Autodesk Fusion 360 part; units mm, degrees
(part 10 of 14)
  spline S90 degree 5 poles (19.8514, 6.85) (19.8445, 6.8509) (19.8307, 6.8527) (19.8101, 6.8553) (19.7826, 6.8588) (19.7482, 6.863) (19.7138, 6.867) (19.6795, 6.8709) (19.6452, 6.8747) (19.6109, 6.8783) (19.5767, 6.8818) (19.5424, 6.8852) (19.5082, 6.8884) (19.474, 6.8915) (19.4399, 6.8944) (19.4057, 6.8972) (19.3716, 6.8999) (19.3376, 6.9024) (19.3035, 6.9048) (19.2695, 6.907) (19.2355, 6.9091) (19.2015, 6.911) (19.1676, 6.9128) (19.1337, 6.9144) (19.0998, 6.9159) (19.066, 6.9173) (19.0322, 6.9185) (18.9984, 6.9195) (18.9647, 6.9204) (18.931, 6.9211) (18.8973, 6.9217) (18.8637, 6.9221) (18.8301, 6.9224) (18.7966, 6.9224) (18.7631, 6.9224) (18.7296, 6.9221) (18.6962, 6.9218) (18.6628, 6.9212) (18.6294, 6.9205) (18.5961, 6.9195) (18.5629, 6.9185) (18.5296, 6.9172) (18.4965, 6.9158) (18.4634, 6.9142) (18.4303, 6.9124) (18.3973, 6.9104) (18.3643, 6.9083) (18.3314, 6.9059) (18.2985, 6.9033) (18.2657, 6.9006) (18.233, 6.8977) (18.2003, 6.8945) (18.1676, 6.8912) (18.1351, 6.8876) (18.1026, 6.8838) (18.0701, 6.8798) (18.0378, 6.8756) (18.0101, 6.8717) (17.9889, 6.8687) (17.9742, 6.8665) (17.9659, 6.8652) (17.9641, 6.8649) knots -1 -1 -1 -1 -1 -1 -0.985714 -0.971429 -0.957143 -0.942857 -0.928571 -0.914286 -0.9 -0.885714 -0.871429 -0.857143 -0.842857 -0.828571 -0.814286 -0.8 -0.785714 -0.771429 -0.757143 -0.742857 -0.728571 -0.714286 -0.7 -0.685714 -0.671429 -0.657143 -0.642857 -0.628571 -0.614286 -0.6 -0.585714 -0.571429 -0.557143 -0.542857 -0.528571 -0.514286 -0.5 -0.485714 -0.471429 -0.457143 -0.442857 -0.428571 -0.414286 -0.4 -0.385714 -0.371429 -0.357143 -0.342857 -0.328571 -0.314286 -0.3 -0.285714 -0.271429 -0.257143 -0.242857 -0.228571 -0.214286 -0.2 -0.195913 -0.195913 -0.195913 -0.195913 -0.195913 -0.195913
  spline S91 degree 3 poles (17.426, 7.1689) (17.4508, 7.1087) (17.4871, 7.0539) (17.5786, 6.9613) (17.633, 6.9244) (17.7354, 6.8809) (17.7803, 6.8688) (17.872, 6.8573) (17.9184, 6.8579) (17.9641, 6.8649) knots 0 0 0 0 0.019532 0.019532 0.039064 0.039064 0.052927 0.052927 0.06679 0.06679 0.06679 0.06679
  arc A46 (17.426, 7.1689) -> (17.3912, 7.2528) centre (0, 0) ccw
  spline S92 degree 3 poles (17.5567, 7.8483) (17.5043, 7.8098) (17.4598, 7.7613) (17.392, 7.6502) (17.3693, 7.5885) (17.3517, 7.4786) (17.3507, 7.4322) (17.3617, 7.3404) (17.3734, 7.2955) (17.3912, 7.2528) knots 0 0 0 0 0.019532 0.019532 0.039064 0.039064 0.052927 0.052927 0.06679 0.06679 0.06679 0.06679
  spline S93 degree 5 poles (17.5567, 7.8483) (17.5582, 7.8494) (17.565, 7.8544) (17.577, 7.8632) (17.5941, 7.876) (17.6164, 7.8929) (17.6423, 7.9127) (17.668, 7.9329) (17.6937, 7.9532) (17.7192, 7.9737) (17.7447, 7.9944) (17.77, 8.0153) (17.7953, 8.0364) (17.8204, 8.0576) (17.8455, 8.079) (17.8704, 8.1006) (17.8952, 8.1224) (17.92, 8.1444) (17.9446, 8.1665) (17.9692, 8.1888) (17.9936, 8.2112) (18.018, 8.2338) (18.0423, 8.2566) (18.0665, 8.2795) (18.0906, 8.3026) (18.1146, 8.3258) (18.1385, 8.3491) (18.1623, 8.3726) (18.1861, 8.3963) (18.2098, 8.4201) (18.2333, 8.444) (18.2568, 8.4681) (18.2802, 8.4923) (18.3035, 8.5166) (18.3267, 8.5411) (18.3499, 8.5657) (18.3729, 8.5905) (18.3959, 8.6153) (18.4188, 8.6403) (18.4416, 8.6655) (18.4644, 8.6907) (18.487, 8.7161) (18.5096, 8.7416) (18.532, 8.7672) (18.5544, 8.793) (18.5768, 8.8189) (18.599, 8.8449) (18.6211, 8.871) (18.6432, 8.8972) (18.6652, 8.9236) (18.6871, 8.95) (18.709, 8.9766) (18.7307, 9.0033) (18.7524, 9.0301) (18.774, 9.0571) (18.7955, 9.0841) (18.8169, 9.1112) (18.8383, 9.1385) (18.8553, 9.1604) (18.868, 9.1769) (18.8765, 9.1879) (18.8807, 9.1934) knots 0.195913 0.195913 0.195913 0.195913 0.195913 0.195913 0.2 0.214286 0.228571 0.242857 0.257143 0.271429 0.285714 0.3 0.314286 0.328571 0.342857 0.357143 0.371429 0.385714 0.4 0.414286 0.428571 0.442857 0.457143 0.471429 0.485714 0.5 0.514286 0.528571 0.542857 0.557143 0.571429 0.585714 0.6 0.614286 0.628571 0.642857 0.657143 0.671429 0.685714 0.7 0.714286 0.728571 0.742857 0.757143 0.771429 0.785714 0.8 0.814286 0.828571 0.842857 0.857143 0.871429 0.885714 0.9 0.914286 0.928571 0.942857 0.957143 0.971429 0.985714 1 1 1 1 1 1
  arc A47 (18.8807, 9.1934) -> (18.5354, 9.8711) centre (0, 0) ccw
  spline S94 degree 5 poles (18.5354, 9.8711) (18.5285, 9.8709) (18.5146, 9.8705) (18.4938, 9.8699) (18.4661, 9.869) (18.4315, 9.8678) (18.3969, 9.8664) (18.3624, 9.8649) (18.3279, 9.8632) (18.2935, 9.8614) (18.2591, 9.8595) (18.2247, 9.8575) (18.1905, 9.8553) (18.1562, 9.853) (18.122, 9.8506) (18.0879, 9.848) (18.0538, 9.8453) (18.0197, 9.8425) (17.9857, 9.8395) (17.9518, 9.8364) (17.9179, 9.8331) (17.884, 9.8297) (17.8502, 9.8262) (17.8165, 9.8225) (17.7828, 9.8187) (17.7492, 9.8147) (17.7156, 9.8106) (17.6821, 9.8063) (17.6486, 9.8019) (17.6152, 9.7974) (17.5819, 9.7927) (17.5486, 9.7878) (17.5154, 9.7828) (17.4822, 9.7777) (17.4492, 9.7723) (17.4161, 9.7669) (17.3832, 9.7613) (17.3503, 9.7555) (17.3175, 9.7495) (17.2847, 9.7434) (17.252, 9.7372) (17.2194, 9.7307) (17.1869, 9.7241) (17.1544, 9.7174) (17.122, 9.7104) (17.0897, 9.7033) (17.0575, 9.696) (17.0254, 9.6885) (16.9933, 9.6809) (16.9613, 9.673) (16.9295, 9.665) (16.8977, 9.6568) (16.866, 9.6484) (16.8343, 9.6397) (16.8028, 9.6309) (16.7714, 9.6219) (16.7401, 9.6127) (16.7134, 9.6045) (16.6929, 9.5982) (16.6788, 9.5937) (16.6708, 9.5912) (16.669, 9.5906) knots -1 -1 -1 -1 -1 -1 -0.985714 -0.971429 -0.957143 -0.942857 -0.928571 -0.914286 -0.9 -0.885714 -0.871429 -0.857143 -0.842857 -0.828571 -0.814286 -0.8 -0.785714 -0.771429 -0.757143 -0.742857 -0.728571 -0.714286 -0.7 -0.685714 -0.671429 -0.657143 -0.642857 -0.628571 -0.614286 -0.6 -0.585714 -0.571429 -0.557143 -0.542857 -0.528571 -0.514286 -0.5 -0.485714 -0.471429 -0.457143 -0.442857 -0.428571 -0.414286 -0.4 -0.385714 -0.371429 -0.357143 -0.342857 -0.328571 -0.314286 -0.3 -0.285714 -0.271429 -0.257143 -0.242857 -0.228571 -0.214286 -0.2 -0.195913 -0.195913 -0.195913 -0.195913 -0.195913 -0.195913
  spline S95 degree 3 poles (16.09, 9.8067) (16.1239, 9.7511) (16.1683, 9.7026) (16.2732, 9.6255) (16.3327, 9.5976) (16.4407, 9.5706) (16.4869, 9.5657) (16.5792, 9.5687) (16.625, 9.5765) (16.669, 9.5906) knots 0 0 0 0 0.019532 0.019532 0.039064 0.039064 0.052927 0.052927 0.06679 0.06679 0.06679 0.06679
  arc A48 (16.09, 9.8067) -> (16.0425, 9.8841) centre (0, 0) ccw
  spline S96 degree 3 poles (16.1129, 10.4982) (16.067, 10.4519) (16.0307, 10.3971) (15.9811, 10.2767) (15.9683, 10.2122) (15.9681, 10.1009) (15.9745, 10.0549) (15.9996, 9.966) (16.0183, 9.9235) (16.0425, 9.8841) knots 0 0 0 0 0.019532 0.019532 0.039064 0.039064 0.052927 0.052927 0.06679 0.06679 0.06679 0.06679
  spline S97 degree 5 poles (16.1129, 10.4982) (16.1142, 10.4995) (16.12, 10.5054) (16.1305, 10.516) (16.1454, 10.5314) (16.1648, 10.5515) (16.1872, 10.5752) (16.2096, 10.5991) (16.2317, 10.6232) (16.2537, 10.6474) (16.2756, 10.6718) (16.2974, 10.6964) (16.319, 10.7212) (16.3405, 10.7461) (16.3619, 10.7712) (16.3832, 10.7965) (16.4043, 10.8219) (16.4253, 10.8474) (16.4462, 10.8731) (16.4669, 10.899) (16.4876, 10.925) (16.5081, 10.9511) (16.5286, 10.9774) (16.5489, 11.0038) (16.5691, 11.0303) (16.5891, 11.057) (16.6091, 11.0838) (16.629, 11.1108) (16.6487, 11.1378) (16.6684, 11.165) (16.6879, 11.1924) (16.7073, 11.2198) (16.7267, 11.2474) (16.7459, 11.2751) (16.765, 11.3029) (16.784, 11.3308) (16.8029, 11.3589) (16.8217, 11.387) (16.8404, 11.4153) (16.859, 11.4437) (16.8775, 11.4722) (16.8959, 11.5008) (16.9142, 11.5295) (16.9324, 11.5584) (16.9505, 11.5873) (16.9685, 11.6163) (16.9864, 11.6455) (17.0042, 11.6748) (17.0219, 11.7041) (17.0395, 11.7336) (17.057, 11.7632) (17.0744, 11.7928) (17.0917, 11.8226) (17.1089, 11.8525) (17.126, 11.8824) (17.143, 11.9125) (17.1599, 11.9427) (17.1768, 11.9729) (17.1902, 11.9972) (17.2001, 12.0155) (17.2068, 12.0277) (17.2101, 12.0338) knots 0.195913 0.195913 0.195913 0.195913 0.195913 0.195913 0.2 0.214286 0.228571 0.242857 0.257143 0.271429 0.285714 0.3 0.314286 0.328571 0.342857 0.357143 0.371429 0.385714 0.4 0.414286 0.428571 0.442857 0.457143 0.471429 0.485714 0.5 0.514286 0.528571 0.542857 0.557143 0.571429 0.585714 0.6 0.614286 0.628571 0.642857 0.657143 0.671429 0.685714 0.7 0.714286 0.728571 0.742857 0.757143 0.771429 0.785714 0.8 0.814286 0.828571 0.842857 0.857143 0.871429 0.885714 0.9 0.914286 0.928571 0.942857 0.957143 0.971429 0.985714 1 1 1 1 1 1
  arc A49 (17.2101, 12.0338) -> (16.763, 12.6491) centre (0, 0) ccw
  spline S98 degree 5 poles (16.763, 12.6491) (16.7562, 12.6479) (16.7426, 12.6453) (16.7221, 12.6415) (16.6949, 12.6362) (16.6609, 12.6296) (16.627, 12.6228) (16.5931, 12.6159) (16.5593, 12.6089) (16.5256, 12.6018) (16.4919, 12.5945) (16.4583, 12.5871) (16.4248, 12.5796) (16.3913, 12.572) (16.3579, 12.5642) (16.3246, 12.5563) (16.2913, 12.5483) (16.2582, 12.5402) (16.225, 12.5319) (16.192, 12.5235) (16.159, 12.515) (16.1261, 12.5064) (16.0933, 12.4976) (16.0606, 12.4887) (16.0279, 12.4796) (15.9953, 12.4704) (15.9628, 12.4611) (15.9303, 12.4517) (15.898, 12.4421) (15.8657, 12.4324) (15.8335, 12.4225) (15.8014, 12.4125) (15.7694, 12.4024) (15.7374, 12.3921) (15.7056, 12.3817) (15.6738, 12.3711) (15.6422, 12.3604) (15.6106, 12.3496) (15.5791, 12.3385) (15.5477, 12.3274) (15.5164, 12.3161) (15.4852, 12.3046) (15.4541, 12.293) (15.4231, 12.2813) (15.3922, 12.2693) (15.3614, 12.2573) (15.3307, 12.245) (15.3001, 12.2326) (15.2697, 12.22) (15.2393, 12.2073) (15.2091, 12.1944) (15.179, 12.1813) (15.149, 12.168) (15.1191, 12.1545) (15.0894, 12.1409) (15.0597, 12.1271) (15.0303, 12.113) (15.0051, 12.1008) (14.9859, 12.0914) (14.9726, 12.0847) (14.9651, 12.081) (14.9635, 12.0801) knots -1 -1 -1 -1 -1 -1 -0.985714 -0.971429 -0.957143 -0.942857 -0.928571 -0.914286 -0.9 -0.885714 -0.871429 -0.857143 -0.842857 -0.828571 -0.814286 -0.8 -0.785714 -0.771429 -0.757143 -0.742857 -0.728571 -0.714286 -0.7 -0.685714 -0.671429 -0.657143 -0.642857 -0.628571 -0.614286 -0.6 -0.585714 -0.571429 -0.557143 -0.542857 -0.528571 -0.514286 -0.5 -0.485714 -0.471429 -0.457143 -0.442857 -0.428571 -0.414286 -0.4 -0.385714 -0.371429 -0.357143 -0.342857 -0.328571 -0.314286 -0.3 -0.285714 -0.271429 -0.257143 -0.242857 -0.228571 -0.214286 -0.2 -0.195913 -0.195913 -0.195913 -0.195913 -0.195913 -0.195913
  spline S99 degree 3 poles (14.3578, 12.203) (14.4, 12.1534) (14.4514, 12.1125) (14.5671, 12.0527) (14.6302, 12.0344) (14.7411, 12.0247) (14.7875, 12.027) (14.8782, 12.0444) (14.9222, 12.0594) (14.9635, 12.0801) knots 0 0 0 0 0.019532 0.019532 0.039064 0.039064 0.052927 0.052927 0.06679 0.06679 0.06679 0.06679
  arc A50 (14.3578, 12.203) -> (14.2988, 12.2721) centre (0, 0) ccw
  spline S100 degree 3 poles (14.2722, 12.8895) (14.2342, 12.8366) (14.2069, 12.7769) (14.1767, 12.6502) (14.1742, 12.5845) (14.1914, 12.4745) (14.2049, 12.4301) (14.2436, 12.3462) (14.2687, 12.3071) (14.2988, 12.2721) knots 0 0 0 0 0.019532 0.019532 0.039064 0.039064 0.052927 0.052927 0.06679 0.06679 0.06679 0.06679
  spline S101 degree 5 poles (14.2722, 12.8895) (14.2733, 12.891) (14.2782, 12.8978) (14.2868, 12.9099) (14.2992, 12.9274) (14.3152, 12.9503) (14.3336, 12.9772) (14.3519, 13.0043) (14.37, 13.0316) (14.388, 13.059) (14.4058, 13.0865) (14.4234, 13.1142) (14.4409, 13.1421) (14.4583, 13.17) (14.4755, 13.1982) (14.4925, 13.2264) (14.5094, 13.2548) (14.5262, 13.2833) (14.5428, 13.312) (14.5592, 13.3408) (14.5756, 13.3697) (14.5918, 13.3987) (14.6078, 13.4279) (14.6237, 13.4571) (14.6395, 13.4865) (14.6552, 13.516) (14.6707, 13.5456) (14.6861, 13.5753) (14.7014, 13.6051) (14.7166, 13.6351) (14.7316, 13.6651) (14.7465, 13.6953) (14.7612, 13.7255) (14.7759, 13.7559) (14.7904, 13.7863) (14.8048, 13.8169) (14.8191, 13.8476) (14.8333, 13.8783) (14.8473, 13.9092) (14.8613, 13.9401) (14.8751, 13.9712) (14.8888, 14.0023) (14.9023, 14.0335) (14.9158, 14.0649) (14.9291, 14.0963) (14.9424, 14.1278) (14.9555, 14.1594) (14.9685, 14.1911) (14.9814, 14.2228) (14.9941, 14.2547) (15.0068, 14.2866) (15.0193, 14.3187) (15.0318, 14.3508) (15.0441, 14.383) (15.0563, 14.4152) (15.0684, 14.4476) (15.0804, 14.4801) (15.0923, 14.5126) (15.1017, 14.5387) (15.1087, 14.5583) (15.1134, 14.5713) (15.1157, 14.5779) knots 0.195913 0.195913 0.195913 0.195913 0.195913 0.195913 0.2 0.214286 0.228571 0.242857 0.257143 0.271429 0.285714 0.3 0.314286 0.328571 0.342857 0.357143 0.371429 0.385714 0.4 0.414286 0.428571 0.442857 0.457143 0.471429 0.485714 0.5 0.514286 0.528571 0.542857 0.557143 0.571429 0.585714 0.6 0.614286 0.628571 0.642857 0.657143 0.671429 0.685714 0.7 0.714286 0.728571 0.742857 0.757143 0.771429 0.785714 0.8 0.814286 0.828571 0.842857 0.857143 0.871429 0.885714 0.9 0.914286 0.928571 0.942857 0.957143 0.971429 0.985714 1 1 1 1 1 1
  arc A51 (15.1157, 14.5779) -> (14.5779, 15.1157) centre (0, 0) ccw
  spline S102 degree 5 poles (14.5779, 15.1157) (14.5713, 15.1134) (14.5583, 15.1087) (14.5387, 15.1017) (14.5126, 15.0923) (14.4801, 15.0804) (14.4476, 15.0684) (14.4152, 15.0563) (14.383, 15.0441) (14.3508, 15.0318) (14.3187, 15.0193) (14.2866, 15.0068) (14.2547, 14.9941) (14.2228, 14.9814) (14.1911, 14.9685) (14.1594, 14.9555) (14.1278, 14.9424) (14.0963, 14.9291) (14.0649, 14.9158) (14.0335, 14.9023) (14.0023, 14.8888) (13.9712, 14.8751) (13.9401, 14.8613) (13.9092, 14.8473) (13.8783, 14.8333) (13.8476, 14.8191) (13.8169, 14.8048) (13.7863, 14.7904) (13.7559, 14.7759) (13.7255, 14.7612) (13.6953, 14.7465) (13.6651, 14.7316) (13.6351, 14.7166) (13.6051, 14.7014) (13.5753, 14.6861) (13.5456, 14.6707) (13.516, 14.6552) (13.4865, 14.6395) (13.4571, 14.6237) (13.4279, 14.6078) (13.3987, 14.5918) (13.3697, 14.5756) (13.3408, 14.5592) (13.312, 14.5428) (13.2833, 14.5262) (13.2548, 14.5094) (13.2264, 14.4925) (13.1982, 14.4755) (13.17, 14.4583) (13.1421, 14.4409) (13.1142, 14.4234) (13.0865, 14.4058) (13.059, 14.388) (13.0316, 14.37) (13.0043, 14.3519) (12.9772, 14.3336) (12.9503, 14.3152) (12.9274, 14.2992) (12.9099, 14.2868) (12.8978, 14.2782) (12.891, 14.2733) (12.8895, 14.2722) knots -1 -1 -1 -1 -1 -1 -0.985714 -0.971429 -0.957143 -0.942857 -0.928571 -0.914286 -0.9 -0.885714 -0.871429 -0.857143 -0.842857 -0.828571 -0.814286 -0.8 -0.785714 -0.771429 -0.757143 -0.742857 -0.728571 -0.714286 -0.7 -0.685714 -0.671429 -0.657143 -0.642857 -0.628571 -0.614286 -0.6 -0.585714 -0.571429 -0.557143 -0.542857 -0.528571 -0.514286 -0.5 -0.485714 -0.471429 -0.457143 -0.442857 -0.428571 -0.414286 -0.4 -0.385714 -0.371429 -0.357143 -0.342857 -0.328571 -0.314286 -0.3 -0.285714 -0.271429 -0.257143 -0.242857 -0.228571 -0.214286 -0.2 -0.195913 -0.195913 -0.195913 -0.195913 -0.195913 -0.195913
  spline S103 degree 3 poles (12.2721, 14.2988) (12.3215, 14.2564) (12.3787, 14.224) (12.5023, 14.1831) (12.5675, 14.1749) (12.6785, 14.1826) (12.724, 14.1922) (12.8109, 14.2236) (12.852, 14.2452) (12.8895, 14.2722) knots 0 0 0 0 0.019532 0.019532 0.039064 0.039064 0.052927 0.052927 0.06679 0.06679 0.06679 0.06679
  arc A52 (12.2721, 14.2988) -> (12.203, 14.3578) centre (0, 0) ccw
  spline S104 degree 3 poles (12.0801, 14.9635) (12.0509, 14.9053) (12.0332, 14.842) (12.0233, 14.7122) (12.031, 14.6469) (12.0652, 14.541) (12.0855, 14.4992) (12.1369, 14.4224) (12.1678, 14.3877) (12.203, 14.3578) knots 0 0 0 0 0.019532 0.019532 0.039064 0.039064 0.052927 0.052927 0.06679 0.06679 0.06679 0.06679
  spline S105 degree 5 poles (12.0801, 14.9635) (12.081, 14.9651) (12.0847, 14.9726) (12.0914, 14.9859) (12.1008, 15.0051) (12.113, 15.0303) (12.1271, 15.0597) (12.1409, 15.0894) (12.1545, 15.1191) (12.168, 15.149) (12.1813, 15.179) (12.1944, 15.2091) (12.2073, 15.2393) (12.22, 15.2697) (12.2326, 15.3001) (12.245, 15.3307) (12.2573, 15.3614) (12.2693, 15.3922) (12.2813, 15.4231) (12.293, 15.4541) (12.3046, 15.4852) (12.3161, 15.5164) (12.3274, 15.5477) (12.3385, 15.5791) (12.3496, 15.6106) (12.3604, 15.6422) (12.3711, 15.6738) (12.3817, 15.7056) (12.3921, 15.7374) (12.4024, 15.7694) (12.4125, 15.8014) (12.4225, 15.8335) (12.4324, 15.8657) (12.4421, 15.898) (12.4517, 15.9303) (12.4611, 15.9628) (12.4704, 15.9953) (12.4796, 16.0279) (12.4887, 16.0606) (12.4976, 16.0933) (12.5064, 16.1261) (12.515, 16.159) (12.5235, 16.192) (12.5319, 16.225) (12.5402, 16.2582) (12.5483, 16.2913) (12.5563, 16.3246) (12.5642, 16.3579) (12.572, 16.3913) (12.5796, 16.4248) (12.5871, 16.4583) (12.5945, 16.4919) (12.6018, 16.5256) (12.6089, 16.5593) (12.6159, 16.5931) (12.6228, 16.627) (12.6296, 16.6609) (12.6362, 16.6949) (12.6415, 16.7221) (12.6453, 16.7426) (12.6479, 16.7562) (12.6491, 16.763) knots 0.195913 0.195913 0.195913 0.195913 0.195913 0.195913 0.2 0.214286 0.228571 0.242857 0.257143 0.271429 0.285714 0.3 0.314286 0.328571 0.342857 0.357143 0.371429 0.385714 0.4 0.414286 0.428571 0.442857 0.457143 0.471429 0.485714 0.5 0.514286 0.528571 0.542857 0.557143 0.571429 0.585714 0.6 0.614286 0.628571 0.642857 0.657143 0.671429 0.685714 0.7 0.714286 0.728571 0.742857 0.757143 0.771429 0.785714 0.8 0.814286 0.828571 0.842857 0.857143 0.871429 0.885714 0.9 0.914286 0.928571 0.942857 0.957143 0.971429 0.985714 1 1 1 1 1 1
  arc A53 (12.6491, 16.763) -> (12.0338, 17.2101) centre (0, 0) ccw
  spline S106 degree 5 poles (12.0338, 17.2101) (12.0277, 17.2068) (12.0155, 17.2001) (11.9972, 17.1902) (11.9729, 17.1768) (11.9427, 17.1599) (11.9125, 17.143) (11.8824, 17.126) (11.8525, 17.1089) (11.8226, 17.0917) (11.7928, 17.0744) (11.7632, 17.057) (11.7336, 17.0395) (11.7041, 17.0219) (11.6748, 17.0042) (11.6455, 16.9864) (11.6163, 16.9685) (11.5873, 16.9505) (11.5584, 16.9324) (11.5295, 16.9142) (11.5008, 16.8959) (11.4722, 16.8775) (11.4437, 16.859) (11.4153, 16.8404) (11.387, 16.8217) (11.3589, 16.8029) (11.3308, 16.784) (11.3029, 16.765) (11.2751, 16.7459) (11.2474, 16.7267) (11.2198, 16.7073) (11.1924, 16.6879) (11.165, 16.6684) (11.1378, 16.6487) (11.1108, 16.629) (11.0838, 16.6091) (11.057, 16.5891) (11.0303, 16.5691) (11.0038, 16.5489) (10.9774, 16.5286) (10.9511, 16.5081) (10.925, 16.4876) (10.899, 16.4669) (10.8731, 16.4462) (10.8474, 16.4253) (10.8219, 16.4043) (10.7965, 16.3832) (10.7712, 16.3619) (10.7461, 16.3405) (10.7212, 16.319) (10.6964, 16.2974) (10.6718, 16.2756) (10.6474, 16.2537) (10.6232, 16.2317) (10.5991, 16.2096) (10.5752, 16.1872) (10.5515, 16.1648) (10.5314, 16.1454) (10.516, 16.1305) (10.5054, 16.12) (10.4995, 16.1142) (10.4982, 16.1129) knots -1 -1 -1 -1 -1 -1 -0.985714 -0.971429 -0.957143 -0.942857 -0.928571 -0.914286 -0.9 -0.885714 -0.871429 -0.857143 -0.842857 -0.828571 -0.814286 -0.8 -0.785714 -0.771429 -0.757143 -0.742857 -0.728571 -0.714286 -0.7 -0.685714 -0.671429 -0.657143 -0.642857 -0.628571 -0.614286 -0.6 -0.585714 -0.571429 -0.557143 -0.542857 -0.528571 -0.514286 -0.5 -0.485714 -0.471429 -0.457143 -0.442857 -0.428571 -0.414286 -0.4 -0.385714 -0.371429 -0.357143 -0.342857 -0.328571 -0.314286 -0.3 -0.285714 -0.271429 -0.257143 -0.242857 -0.228571 -0.214286 -0.2 -0.195913 -0.195913 -0.195913 -0.195913 -0.195913 -0.195913
  spline S107 degree 3 poles (9.8841, 16.0425) (9.9396, 16.0084) (10.0011, 15.9854) (10.1296, 15.9643) (10.1953, 15.9664) (10.3038, 15.9914) (10.3472, 16.008) (10.4281, 16.0525) (10.4653, 16.0803) (10.4982, 16.1129) knots 0 0 0 0 0.019532 0.019532 0.039064 0.039064 0.052927 0.052927 0.06679 0.06679 0.06679 0.06679
  arc A54 (9.8841, 16.0425) -> (9.8067, 16.09) centre (0, 0) ccw
  spline S108 degree 3 poles (9.5906, 16.669) (9.5708, 16.607) (9.5633, 16.5417) (9.5737, 16.4119) (9.5916, 16.3486) (9.642, 16.2494) (9.6685, 16.2113) (9.7313, 16.1434) (9.7672, 16.114) (9.8067, 16.09) knots 0 0 0 0 0.019532 0.019532 0.039064 0.039064 0.052927 0.052927 0.06679 0.06679 0.06679 0.06679
  spline S109 degree 5 poles (9.5906, 16.669) (9.5912, 16.6708) (9.5937, 16.6788) (9.5982, 16.6929) (9.6045, 16.7134) (9.6127, 16.7401) (9.6219, 16.7714) (9.6309, 16.8028) (9.6397, 16.8343) (9.6484, 16.866) (9.6568, 16.8977) (9.665, 16.9295) (9.673, 16.9613) (9.6809, 16.9933) (9.6885, 17.0254) (9.696, 17.0575) (9.7033, 17.0897) (9.7104, 17.122) (9.7174, 17.1544) (9.7241, 17.1869) (9.7307, 17.2194) (9.7372, 17.252) (9.7434, 17.2847) (9.7495, 17.3175) (9.7555, 17.3503) (9.7613, 17.3832) (9.7669, 17.4161) (9.7723, 17.4492) (9.7777, 17.4822) (9.7828, 17.5154) (9.7878, 17.5486) (9.7927, 17.5819) (9.7974, 17.6152) (9.8019, 17.6486) (9.8063, 17.6821) (9.8106, 17.7156) (9.8147, 17.7492) (9.8187, 17.7828) (9.8225, 17.8165) (9.8262, 17.8502) (9.8297, 17.884) (9.8331, 17.9179) (9.8364, 17.9518) (9.8395, 17.9857) (9.8425, 18.0197) (9.8453, 18.0538) (9.848, 18.0879) (9.8506, 18.122) (9.853, 18.1562) (9.8553, 18.1905) (9.8575, 18.2247) (9.8595, 18.2591) (9.8614, 18.2935) (9.8632, 18.3279) (9.8649, 18.3624) (9.8664, 18.3969) (9.8678, 18.4315) (9.869, 18.4661) (9.8699, 18.4938) (9.8705, 18.5146) (9.8709, 18.5285) (9.8711, 18.5354) knots 0.195913 0.195913 0.195913 0.195913 0.195913 0.195913 0.2 0.214286 0.228571 0.242857 0.257143 0.271429 0.285714 0.3 0.314286 0.328571 0.342857 0.357143 0.371429 0.385714 0.4 0.414286 0.428571 0.442857 0.457143 0.471429 0.485714 0.5 0.514286 0.528571 0.542857 0.557143 0.571429 0.585714 0.6 0.614286 0.628571 0.642857 0.657143 0.671429 0.685714 0.7 0.714286 0.728571 0.742857 0.757143 0.771429 0.785714 0.8 0.814286 0.828571 0.842857 0.857143 0.871429 0.885714 0.9 0.914286 0.928571 0.942857 0.957143 0.971429 0.985714 1 1 1 1 1 1
  arc A55 (9.8711, 18.5354) -> (9.1934, 18.8807) centre (0, 0) ccw
  spline S110 degree 5 poles (9.1934, 18.8807) (9.1879, 18.8765) (9.1769, 18.868) (9.1604, 18.8553) (9.1385, 18.8383) (9.1112, 18.8169) (9.0841, 18.7955) (9.0571, 18.774) (9.0301, 18.7524) (9.0033, 18.7307) (8.9766, 18.709) (8.95, 18.6871) (8.9236, 18.6652) (8.8972, 18.6432) (8.871, 18.6211) (8.8449, 18.599) (8.8189, 18.5768) (8.793, 18.5544) (8.7672, 18.532) (8.7416, 18.5096) (8.7161, 18.487) (8.6907, 18.4644) (8.6655, 18.4416) (8.6403, 18.4188) (8.6153, 18.3959) (8.5905, 18.3729) (8.5657, 18.3499) (8.5411, 18.3267) (8.5166, 18.3035) (8.4923, 18.2802) (8.4681, 18.2568) (8.444, 18.2333) (8.4201, 18.2098) (8.3963, 18.1861) (8.3726, 18.1623) (8.3491, 18.1385) (8.3258, 18.1146) (8.3026, 18.0906) (8.2795, 18.0665) (8.2566, 18.0423) (8.2338, 18.018) (8.2112, 17.9936) (8.1888, 17.9692) (8.1665, 17.9446) (8.1444, 17.92) (8.1224, 17.8952) (8.1006, 17.8704) (8.079, 17.8455) (8.0576, 17.8204) (8.0364, 17.7953) (8.0153, 17.77) (7.9944, 17.7447) (7.9737, 17.7192) (7.9532, 17.6937) (7.9329, 17.668) (7.9127, 17.6423) (7.8929, 17.6164) (7.876, 17.5941) (7.8632, 17.577) (7.8544, 17.565) (7.8494, 17.5582) (7.8483, 17.5567) knots -1 -1 -1 -1 -1 -1 -0.985714 -0.971429 -0.957143 -0.942857 -0.928571 -0.914286 -0.9 -0.885714 -0.871429 -0.857143 -0.842857 -0.828571 -0.814286 -0.8 -0.785714 -0.771429 -0.757143 -0.742857 -0.728571 -0.714286 -0.7 -0.685714 -0.671429 -0.657143 -0.642857 -0.628571 -0.614286 -0.6 -0.585714 -0.571429 -0.557143 -0.542857 -0.528571 -0.514286 -0.5 -0.485714 -0.471429 -0.457143 -0.442857 -0.428571 -0.414286 -0.4 -0.385714 -0.371429 -0.357143 -0.342857 -0.328571 -0.314286 -0.3 -0.285714 -0.271429 -0.257143 -0.242857 -0.228571 -0.214286 -0.2 -0.195913 -0.195913 -0.195913 -0.195913 -0.195913 -0.195913
  spline S111 degree 3 poles (7.2528, 17.3912) (7.3129, 17.3662) (7.3774, 17.3531) (7.5076, 17.3523) (7.5721, 17.3647) (7.6753, 17.4064) (7.7156, 17.4295) (7.7886, 17.4862) (7.821, 17.5195) (7.8483, 17.5567) knots 0 0 0 0 0.019532 0.019532 0.039064 0.039064 0.052927 0.052927 0.06679 0.06679 0.06679 0.06679
  arc A56 (7.2528, 17.3912) -> (7.1689, 17.426) centre (0, 0) ccw
  spline S112 degree 3 poles (6.8649, 17.9641) (6.8551, 17.8997) (6.8579, 17.8341) (6.8885, 17.7075) (6.916, 17.6478) (6.9813, 17.5577) (7.0135, 17.5242) (7.0861, 17.467) (7.1262, 17.4436) (7.1689, 17.426) knots 0 0 0 0 0.019532 0.019532 0.039064 0.039064 0.052927 0.052927 0.06679 0.06679 0.06679 0.06679
  spline S113 degree 5 poles (6.8649, 17.9641) (6.8652, 17.9659) (6.8665, 17.9742) (6.8687, 17.9889) (6.8717, 18.0101) (6.8756, 18.0378) (6.8798, 18.0701) (6.8838, 18.1026) (6.8876, 18.1351) (6.8912, 18.1676) (6.8945, 18.2003) (6.8977, 18.233) (6.9006, 18.2657) (6.9033, 18.2985) (6.9059, 18.3314) (6.9083, 18.3643) (6.9104, 18.3973) (6.9124, 18.4303) (6.9142, 18.4634) (6.9158, 18.4965) (6.9172, 18.5296) (6.9185, 18.5629) (6.9195, 18.5961) (6.9205, 18.6294) (6.9212, 18.6628) (6.9218, 18.6962) (6.9221, 18.7296) (6.9224, 18.7631) (6.9224, 18.7966) (6.9224, 18.8301) (6.9221, 18.8637) (6.9217, 18.8973) (6.9211, 18.931) (6.9204, 18.9647) (6.9195, 18.9984) (6.9185, 19.0322) (6.9173, 19.066) (6.9159, 19.0998) (6.9144, 19.1337) (6.9128, 19.1676) (6.911, 19.2015) (6.9091, 19.2355) (6.907, 19.2695) (6.9048, 19.3035) (6.9024, 19.3376) (6.8999, 19.3716) (6.8972, 19.4057) (6.8944, 19.4399) (6.8915, 19.474) (6.8884, 19.5082) (6.8852, 19.5424) (6.8818, 19.5767) (6.8783, 19.6109) (6.8747, 19.6452) (6.8709, 19.6795) (6.867, 19.7138) (6.863, 19.7482) (6.8588, 19.7826) (6.8553, 19.8101) (6.8527, 19.8307) (6.8509, 19.8445) (6.85, 19.8514) knots 0.195913 0.195913 0.195913 0.195913 0.195913 0.195913 0.2 0.214286 0.228571 0.242857 0.257143 0.271429 0.285714 0.3 0.314286 0.328571 0.342857 0.357143 0.371429 0.385714 0.4 0.414286 0.428571 0.442857 0.457143 0.471429 0.485714 0.5 0.514286 0.528571 0.542857 0.557143 0.571429 0.585714 0.6 0.614286 0.628571 0.642857 0.657143 0.671429 0.685714 0.7 0.714286 0.728571 0.742857 0.757143 0.771429 0.785714 0.8 0.814286 0.828571 0.842857 0.857143 0.871429 0.885714 0.9 0.914286 0.928571 0.942857 0.957143 0.971429 0.985714 1 1 1 1 1 1
  arc A57 (6.85, 19.8514) -> (6.1266, 20.0864) centre (0, 0) ccw
  spline S114 degree 5 poles (6.1266, 20.0864) (6.1218, 20.0814) (6.1123, 20.0713) (6.098, 20.0562) (6.079, 20.0359) (6.0555, 20.0106) (6.032, 19.9851) (6.0087, 19.9597) (5.9854, 19.9341) (5.9623, 19.9085) (5.9394, 19.8829) (5.9165, 19.8571) (5.8938, 19.8314) (5.8712, 19.8055) (5.8488, 19.7796) (5.8265, 19.7536) (5.8043, 19.7276) (5.7822, 19.7015) (5.7603, 19.6754) (5.7385, 19.6492) (5.7168, 19.6229) (5.6953, 19.5966) (5.6739, 19.5702) (5.6526, 19.5437) (5.6315, 19.5172) (5.6105, 19.4906) (5.5897, 19.4639) (5.569, 19.4372) (5.5485, 19.4105) (5.5281, 19.3836) (5.5078, 19.3567) (5.4877, 19.3298) (5.4678, 19.3027) (5.448, 19.2757) (5.4283, 19.2485) (5.4088, 19.2213) (5.3895, 19.194) (5.3703, 19.1667) (5.3513, 19.1393) (5.3325, 19.1118) (5.3138, 19.0842) (5.2953, 19.0566) (5.277, 19.029) (5.2588, 19.0012) (5.2408, 18.9734) (5.223, 18.9455) (5.2054, 18.9176) (5.1879, 18.8896) (5.1707, 18.8615) (5.1536, 18.8333) (5.1368, 18.8051) (5.1201, 18.7768) (5.1036, 18.7485) (5.0873, 18.72) (5.0713, 18.6915) (5.0555, 18.6629) (5.0399, 18.6342) (5.0267, 18.6096) (5.0168, 18.5906) (5.0099, 18.5774) (5.006, 18.57) (5.0052, 18.5683) knots -1 -1 -1 -1 -1 -1 -0.985714 -0.971429 -0.957143 -0.942857 -0.928571 -0.914286 -0.9 -0.885714 -0.871429 -0.857143 -0.842857 -0.828571 -0.814286 -0.8 -0.785714 -0.771429 -0.757143 -0.742857 -0.728571 -0.714286 -0.7 -0.685714 -0.671429 -0.657143 -0.642857 -0.628571 -0.614286 -0.6 -0.585714 -0.571429 -0.557143 -0.542857 -0.528571 -0.514286 -0.5 -0.485714 -0.471429 -0.457143 -0.442857 -0.428571 -0.414286 -0.4 -0.385714 -0.371429 -0.357143 -0.342857 -0.328571 -0.314286 -0.3 -0.285714 -0.271429 -0.257143 -0.242857 -0.228571 -0.214286 -0.2 -0.195913 -0.195913 -0.195913 -0.195913 -0.195913 -0.195913
  spline S115 degree 3 poles (4.443, 18.3117) (4.5062, 18.2964) (4.5719, 18.2935) (4.7006, 18.3131) (4.7625, 18.3354) (4.8579, 18.3928) (4.894, 18.4219) (4.9572, 18.4893) (4.984, 18.5273) (5.0052, 18.5683) knots 0 0 0 0 0.019532 0.019532 0.039064 0.039064 0.052927 0.052927 0.06679 0.06679 0.06679 0.06679
  arc A58 (4.443, 18.3117) -> (4.3546, 18.3329) centre (0, 0) ccw
  spline S116 degree 3 poles (3.9702, 18.8168) (3.9705, 18.7517) (3.9836, 18.6873) (4.0336, 18.5671) (4.0701, 18.5124) (4.1487, 18.4336) (4.1858, 18.4056) (4.2664, 18.3605) (4.3097, 18.3436) (4.3546, 18.3329) knots 0 0 0 0 0.019532 0.019532 0.039064 0.039064 0.052927 0.052927 0.06679 0.06679 0.06679 0.06679
  spline S117 degree 5 poles (3.9702, 18.8168) (3.9702, 18.8187) (3.9701, 18.8271) (3.97, 18.8419) (3.9697, 18.8633) (3.9692, 18.8913) (3.9683, 18.9239) (3.9672, 18.9566) (3.9658, 18.9893) (3.9643, 19.022) (3.9625, 19.0547) (3.9605, 19.0875) (3.9583, 19.1203) (3.9558, 19.1532) (3.9532, 19.186) (3.9504, 19.2189) (3.9474, 19.2518) (3.9442, 19.2847) (3.9407, 19.3177) (3.9372, 19.3506) (3.9334, 19.3836) (3.9294, 19.4166) (3.9253, 19.4496) (3.921, 19.4827) (3.9165, 19.5157) (3.9118, 19.5488) (3.907, 19.5819) (3.902, 19.615) (3.8968, 19.6481) (3.8914, 19.6812) (3.8859, 19.7143) (3.8803, 19.7475) (3.8744, 19.7806) (3.8684, 19.8138) (3.8623, 19.847) (3.856, 19.8802) (3.8495, 19.9134) (3.8429, 19.9466) (3.8361, 19.9798) (3.8292, 20.013) (3.8221, 20.0463) (3.8149, 20.0795) (3.8075, 20.1127) (3.8, 20.146) (3.7923, 20.1793) (3.7845, 20.2125) (3.7766, 20.2458) (3.7685, 20.2791) (3.7602, 20.3123) (3.7518, 20.3456) (3.7433, 20.3789) (3.7346, 20.4122) (3.7258, 20.4455) (3.7168, 20.4788) (3.7078, 20.5121) (3.6985, 20.5454) (3.6892, 20.5787) (3.6797, 20.612) (3.6719, 20.6386) (3.6661, 20.6586) (3.6622, 20.6719) (3.6602, 20.6786) knots 0.195913 0.195913 0.195913 0.195913 0.195913 0.195913 0.2 0.214286 0.228571 0.242857 0.257143 0.271429 0.285714 0.3 0.314286 0.328571 0.342857 0.357143 0.371429 0.385714 0.4 0.414286 0.428571 0.442857 0.457143 0.471429 0.485714 0.5 0.514286 0.528571 0.542857 0.557143 0.571429 0.585714 0.6 0.614286 0.628571 0.642857 0.657143 0.671429 0.685714 0.7 0.714286 0.728571 0.742857 0.757143 0.771429 0.785714 0.8 0.814286 0.828571 0.842857 0.857143 0.871429 0.885714 0.9 0.914286 0.928571 0.942857 0.957143 0.971429 0.985714 1 1 1 1 1 1
  arc A59 (3.6602, 20.6786) -> (2.909, 20.7975) centre (0, 0) ccw
  spline S118 degree 5 poles (2.909, 20.7975) (2.905, 20.7918) (2.8972, 20.7804) (2.8854, 20.7632) (2.8699, 20.7402) (2.8506, 20.7115) (2.8314, 20.6827) (2.8123, 20.6539) (2.7934, 20.625) (2.7746, 20.5961) (2.7559, 20.5672) (2.7374, 20.5382) (2.719, 20.5092) (2.7007, 20.4801) (2.6826, 20.451) (2.6646, 20.4219) (2.6467, 20.3927) (2.629, 20.3635) (2.6114, 20.3342) (2.594, 20.3049) (2.5767, 20.2756) (2.5596, 20.2462) (2.5426, 20.2168) (2.5257, 20.1873) (2.509, 20.1578) (2.4925, 20.1283) (2.476, 20.0987) (2.4598, 20.0691) (2.4437, 20.0395) (2.4277, 20.0098) (2.4119, 19.98) (2.3963, 19.9503) (2.3808, 19.9204) (2.3655, 19.8906) (2.3504, 19.8607) (2.3354, 19.8308) (2.3206, 19.8008) (2.3059, 19.7708) (2.2914, 19.7408) (2.2771, 19.7107) (2.263, 19.6805) (2.249, 19.6504) (2.2352, 19.6202) (2.2216, 19.5899) (2.2082, 19.5597) (2.195, 19.5293) (2.1819, 19.499) (2.1691, 19.4686) (2.1564, 19.4382) (2.144, 19.4077) (2.1317, 19.3772) (2.1197, 19.3466) (2.1079, 19.316) (2.0963, 19.2854) (2.0849, 19.2547) (2.0737, 19.224) (2.0628, 19.1932) (2.0536, 19.1668) (2.0468, 19.1465) (2.0421, 19.1324) (2.0394, 19.1245) (2.0388, 19.1227) knots -1 -1 -1 -1 -1 -1 -0.985714 -0.971429 -0.957143 -0.942857 -0.928571 -0.914286 -0.9 -0.885714 -0.871429 -0.857143 -0.842857 -0.828571 -0.814286 -0.8 -0.785714 -0.771429 -0.757143 -0.742857 -0.728571 -0.714286 -0.7 -0.685714 -0.671429 -0.657143 -0.642857 -0.628571 -0.614286 -0.6 -0.585714 -0.571429 -0.557143 -0.542857 -0.528571 -0.514286 -0.5 -0.485714 -0.471429 -0.457143 -0.442857 -0.428571 -0.414286 -0.4 -0.385714 -0.371429 -0.357143 -0.342857 -0.328571 -0.314286 -0.3 -0.285714 -0.271429 -0.257143 -0.242857 -0.228571 -0.214286 -0.2 -0.195913 -0.195913 -0.195913 -0.195913 -0.195913 -0.195913
  spline S119 degree 3 poles (1.5237, 18.7813) (1.5886, 18.776) (1.6539, 18.7835) (1.7779, 18.823) (1.8355, 18.8547) (1.9208, 18.9263) (1.9519, 18.9607) (2.0038, 19.0372) (2.0243, 19.0788) (2.0388, 19.1227) knots 0 0 0 0 0.019532 0.019532 0.039064 0.039064 0.052927 0.052927 0.06679 0.06679 0.06679 0.06679
  arc A60 (1.5237, 18.7813) -> (1.4331, 18.7884) centre (0, 0) ccw
  spline S120 degree 3 poles (0.9777, 19.2062) (0.9882, 19.142) (1.0112, 19.0804) (1.0794, 18.9695) (1.1241, 18.9212) (1.214, 18.8557) (1.255, 18.8338) (1.3417, 18.8018) (1.387, 18.7919) (1.4331, 18.7884) knots 0 0 0 0 0.019532 0.019532 0.039064 0.039064 0.052927 0.052927 0.06679 0.06679 0.06679 0.06679
  spline S121 degree 5 poles (0.9777, 19.2062) (0.9774, 19.2081) (0.9761, 19.2163) (0.9736, 19.231) (0.97, 19.2521) (0.9651, 19.2796) (0.9591, 19.3117) (0.9529, 19.3438) (0.9464, 19.3759) (0.9398, 19.4079) (0.9329, 19.44) (0.9258, 19.4721) (0.9184, 19.5041) (0.9109, 19.5362) (0.9032, 19.5682) (0.8953, 19.6003) (0.8871, 19.6323) (0.8788, 19.6643) (0.8703, 19.6963) (0.8616, 19.7283) (0.8527, 19.7603) (0.8436, 19.7923) (0.8344, 19.8242) (0.8249, 19.8562) (0.8153, 19.8881) (0.8055, 19.92) (0.7956, 19.952) (0.7855, 19.9839) (0.7752, 20.0158) (0.7647, 20.0476) (0.7541, 20.0795) (0.7433, 20.1114) (0.7324, 20.1432) (0.7213, 20.175) (0.71, 20.2068) (0.6986, 20.2386) (0.687, 20.2704) (0.6753, 20.3022) (0.6634, 20.3339) (0.6513, 20.3656) (0.6392, 20.3974) (0.6268, 20.4291) (0.6143, 20.4607) (0.6017, 20.4924) (0.5889, 20.5241) (0.576, 20.5557) (0.5629, 20.5873) (0.5497, 20.6189) (0.5364, 20.6505) (0.5229, 20.682) (0.5092, 20.7136) (0.4955, 20.7451) (0.4815, 20.7766) (0.4675, 20.8081) (0.4533, 20.8396) (0.439, 20.871) (0.4245, 20.9024) (0.4099, 20.9338) (0.3982, 20.9589) (0.3893, 20.9777) (0.3833, 20.9903) (0.3803, 20.9966) knots 0.195913 0.195913 0.195913 0.195913 0.195913 0.195913 0.2 0.214286 0.228571 0.242857 0.257143 0.271429 0.285714 0.3 0.314286 0.328571 0.342857 0.357143 0.371429 0.385714 0.4 0.414286 0.428571 0.442857 0.457143 0.471429 0.485714 0.5 0.514286 0.528571 0.542857 0.557143 0.571429 0.585714 0.6 0.614286 0.628571 0.642857 0.657143 0.671429 0.685714 0.7 0.714286 0.728571 0.742857 0.757143 0.771429 0.785714 0.8 0.814286 0.828571 0.842857 0.857143 0.871429 0.885714 0.9 0.914286 0.928571 0.942857 0.957143 0.971429 0.985714 1 1 1 1 1 1
  arc A61 (0.3803, 20.9966) -> (-0.3803, 20.9966) centre (0, 0) ccw
  spline S122 degree 5 poles (-0.3803, 20.9966) (-0.3833, 20.9903) (-0.3893, 20.9777) (-0.3982, 20.9589) (-0.4099, 20.9338) (-0.4245, 20.9024) (-0.439, 20.871) (-0.4533, 20.8396) (-0.4675, 20.8081) (-0.4815, 20.7766) (-0.4955, 20.7451) (-0.5092, 20.7136) (-0.5229, 20.682) (-0.5364, 20.6505) (-0.5497, 20.6189) (-0.5629, 20.5873) (-0.576, 20.5557) (-0.5889, 20.5241) (-0.6017, 20.4924) (-0.6143, 20.4607) (-0.6268, 20.4291) (-0.6392, 20.3974) (-0.6513, 20.3656) (-0.6634, 20.3339) (-0.6753, 20.3022) (-0.687, 20.2704) (-0.6986, 20.2386) (-0.71, 20.2068) (-0.7213, 20.175) (-0.7324, 20.1432) (-0.7433, 20.1114) (-0.7541, 20.0795) (-0.7647, 20.0476) (-0.7752, 20.0158) (-0.7855, 19.9839) (-0.7956, 19.952) (-0.8055, 19.92) (-0.8153, 19.8881) (-0.8249, 19.8562) (-0.8344, 19.8242) (-0.8436, 19.7923) (-0.8527, 19.7603) (-0.8616, 19.7283) (-0.8703, 19.6963) (-0.8788, 19.6643) (-0.8871, 19.6323) (-0.8953, 19.6003) (-0.9032, 19.5682) (-0.9109, 19.5362) (-0.9184, 19.5041) (-0.9258, 19.4721) (-0.9329, 19.44) (-0.9398, 19.4079) (-0.9464, 19.3759) (-0.9529, 19.3438) (-0.9591, 19.3117) (-0.9651, 19.2796) (-0.97, 19.2521) (-0.9736, 19.231) (-0.9761, 19.2163) (-0.9774, 19.2081) (-0.9777, 19.2062) knots -1 -1 -1 -1 -1 -1 -0.985714 -0.971429 -0.957143 -0.942857 -0.928571 -0.914286 -0.9 -0.885714 -0.871429 -0.857143 -0.842857 -0.828571 -0.814286 -0.8 -0.785714 -0.771429 -0.757143 -0.742857 -0.728571 -0.714286 -0.7 -0.685714 -0.671429 -0.657143 -0.642857 -0.628571 -0.614286 -0.6 -0.585714 -0.571429 -0.557143 -0.542857 -0.528571 -0.514286 -0.5 -0.485714 -0.471429 -0.457143 -0.442857 -0.428571 -0.414286 -0.4 -0.385714 -0.371429 -0.357143 -0.342857 -0.328571 -0.314286 -0.3 -0.285714 -0.271429 -0.257143 -0.242857 -0.228571 -0.214286 -0.2 -0.195913 -0.195913 -0.195913 -0.195913 -0.195913 -0.195913
  spline S123 degree 3 poles (-1.4331, 18.7884) (-1.3682, 18.7934) (-1.3049, 18.811) (-1.1885, 18.8694) (-1.1366, 18.9097) (-1.0635, 18.9937) (-1.0382, 19.0326) (-0.9989, 19.1163) (-0.9852, 19.1606) (-0.9777, 19.2062) knots 0 0 0 0 0.019532 0.019532 0.039064 0.039064 0.052927 0.052927 0.06679 0.06679 0.06679 0.06679
  arc A62 (-1.4331, 18.7884) -> (-1.5237, 18.7813) centre (0, 0) ccw
  spline S124 degree 3 poles (-2.0388, 19.1227) (-2.0184, 19.0609) (-1.9861, 19.0037) (-1.9013, 18.9048) (-1.8497, 18.8641) (-1.7506, 18.8134) (-1.7067, 18.7982) (-1.6161, 18.7802) (-1.5697, 18.7776) (-1.5237, 18.7813) knots 0 0 0 0 0.019532 0.019532 0.039064 0.039064 0.052927 0.052927 0.06679 0.06679 0.06679 0.06679
  spline S125 degree 5 poles (-2.0388, 19.1227) (-2.0394, 19.1245) (-2.0421, 19.1324) (-2.0468, 19.1465) (-2.0536, 19.1668) (-2.0628, 19.1932) (-2.0737, 19.224) (-2.0849, 19.2547) (-2.0963, 19.2854) (-2.1079, 19.316) (-2.1197, 19.3466) (-2.1317, 19.3772) (-2.144, 19.4077) (-2.1564, 19.4382) (-2.1691, 19.4686) (-2.1819, 19.499) (-2.195, 19.5293) (-2.2082, 19.5597) (-2.2216, 19.5899) (-2.2352, 19.6202) (-2.249, 19.6504) (-2.263, 19.6805) (-2.2771, 19.7107) (-2.2914, 19.7408) (-2.3059, 19.7708) (-2.3206, 19.8008) (-2.3354, 19.8308) (-2.3504, 19.8607) (-2.3655, 19.8906) (-2.3808, 19.9204) (-2.3963, 19.9503) (-2.4119, 19.98) (-2.4277, 20.0098) (-2.4437, 20.0395) (-2.4598, 20.0691) (-2.476, 20.0987) (-2.4925, 20.1283) (-2.509, 20.1578) (-2.5257, 20.1873) (-2.5426, 20.2168) (-2.5596, 20.2462) (-2.5767, 20.2756) (-2.594, 20.3049) (-2.6114, 20.3342) (-2.629, 20.3635) (-2.6467, 20.3927) (-2.6646, 20.4219) (-2.6826, 20.451) (-2.7007, 20.4801) (-2.719, 20.5092) (-2.7374, 20.5382) (-2.7559, 20.5672) (-2.7746, 20.5961) (-2.7934, 20.625) (-2.8123, 20.6539) (-2.8314, 20.6827) (-2.8506, 20.7115) (-2.8699, 20.7402) (-2.8854, 20.7632) (-2.8972, 20.7804) (-2.905, 20.7918) (-2.909, 20.7975) knots 0.195913 0.195913 0.195913 0.195913 0.195913 0.195913 0.2 0.214286 0.228571 0.242857 0.257143 0.271429 0.285714 0.3 0.314286 0.328571 0.342857 0.357143 0.371429 0.385714 0.4 0.414286 0.428571 0.442857 0.457143 0.471429 0.485714 0.5 0.514286 0.528571 0.542857 0.557143 0.571429 0.585714 0.6 0.614286 0.628571 0.642857 0.657143 0.671429 0.685714 0.7 0.714286 0.728571 0.742857 0.757143 0.771429 0.785714 0.8 0.814286 0.828571 0.842857 0.857143 0.871429 0.885714 0.9 0.914286 0.928571 0.942857 0.957143 0.971429 0.985714 1 1 1 1 1 1
  arc A63 (-2.909, 20.7975) -> (-3.6602, 20.6786) centre (0, 0) ccw
  spline S126 degree 5 poles (-3.6602, 20.6786) (-3.6622, 20.6719) (-3.6661, 20.6586) (-3.6719, 20.6386) (-3.6797, 20.612) (-3.6892, 20.5787) (-3.6985, 20.5454) (-3.7078, 20.5121) (-3.7168, 20.4788) (-3.7258, 20.4455) (-3.7346, 20.4122) (-3.7433, 20.3789) (-3.7518, 20.3456) (-3.7602, 20.3123) (-3.7685, 20.2791) (-3.7766, 20.2458) (-3.7845, 20.2125) (-3.7923, 20.1793) (-3.8, 20.146) (-3.8075, 20.1127) (-3.8149, 20.0795) (-3.8221, 20.0463) (-3.8292, 20.013) (-3.8361, 19.9798) (-3.8429, 19.9466) (-3.8495, 19.9134) (-3.856, 19.8802) (-3.8623, 19.847) (-3.8684, 19.8138) (-3.8744, 19.7806) (-3.8803, 19.7475) (-3.8859, 19.7143) (-3.8914, 19.6812) (-3.8968, 19.6481) (-3.902, 19.615) (-3.907, 19.5819) (-3.9118, 19.5488) (-3.9165, 19.5157) (-3.921, 19.4827) (-3.9253, 19.4496) (-3.9294, 19.4166) (-3.9334, 19.3836) (-3.9372, 19.3506) (-3.9407, 19.3177) (-3.9442, 19.2847) (-3.9474, 19.2518) (-3.9504, 19.2189) (-3.9532, 19.186) (-3.9558, 19.1532) (-3.9583, 19.1203) (-3.9605, 19.0875) (-3.9625, 19.0547) (-3.9643, 19.022) (-3.9658, 18.9893) (-3.9672, 18.9566) (-3.9683, 18.9239) (-3.9692, 18.8913) (-3.9697, 18.8633) (-3.97, 18.8419) (-3.9701, 18.8271) (-3.9702, 18.8187) (-3.9702, 18.8168) knots -1 -1 -1 -1 -1 -1 -0.985714 -0.971429 -0.957143 -0.942857 -0.928571 -0.914286 -0.9 -0.885714 -0.871429 -0.857143 -0.842857 -0.828571 -0.814286 -0.8 -0.785714 -0.771429 -0.757143 -0.742857 -0.728571 -0.714286 -0.7 -0.685714 -0.671429 -0.657143 -0.642857 -0.628571 -0.614286 -0.6 -0.585714 -0.571429 -0.557143 -0.542857 -0.528571 -0.514286 -0.5 -0.485714 -0.471429 -0.457143 -0.442857 -0.428571 -0.414286 -0.4 -0.385714 -0.371429 -0.357143 -0.342857 -0.328571 -0.314286 -0.3 -0.285714 -0.271429 -0.257143 -0.242857 -0.228571 -0.214286 -0.2 -0.195913 -0.195913 -0.195913 -0.195913 -0.195913 -0.195913
  spline S127 degree 3 poles (-4.3546, 18.3329) (-4.2913, 18.348) (-4.2315, 18.3752) (-4.1257, 18.4512) (-4.0807, 18.4991) (-4.0217, 18.5935) (-4.0028, 18.6359) (-3.9771, 18.7247) (-3.9704, 18.7706) (-3.9702, 18.8168) knots 0 0 0 0 0.019532 0.019532 0.039064 0.039064 0.052927 0.052927 0.06679 0.06679 0.06679 0.06679
  arc A64 (-4.3546, 18.3329) -> (-4.443, 18.3117) centre (0, 0) ccw
  spline S128 degree 3 poles (-5.0052, 18.5683) (-4.9753, 18.5105) (-4.9345, 18.459) (-4.8353, 18.3746) (-4.7779, 18.3425) (-4.6721, 18.308) (-4.6264, 18.2998) (-4.5341, 18.2962) (-4.4879, 18.3008) (-4.443, 18.3117) knots 0 0 0 0 0.019532 0.019532 0.039064 0.039064 0.052927 0.052927 0.06679 0.06679 0.06679 0.06679
  spline S129 degree 5 poles (-5.0052, 18.5683) (-5.006, 18.57) (-5.0099, 18.5774) (-5.0168, 18.5906) (-5.0267, 18.6096) (-5.0399, 18.6342) (-5.0555, 18.6629) (-5.0713, 18.6915) (-5.0873, 18.72) (-5.1036, 18.7485) (-5.1201, 18.7768) (-5.1368, 18.8051) (-5.1536, 18.8333) (-5.1707, 18.8615) (-5.1879, 18.8896) (-5.2054, 18.9176) (-5.223, 18.9455) (-5.2408, 18.9734) (-5.2588, 19.0012) (-5.277, 19.029) (-5.2953, 19.0566) (-5.3138, 19.0842) (-5.3325, 19.1118) (-5.3513, 19.1393) (-5.3703, 19.1667) (-5.3895, 19.194) (-5.4088, 19.2213) (-5.4283, 19.2485) (-5.448, 19.2757) (-5.4678, 19.3027) (-5.4877, 19.3298) (-5.5078, 19.3567) (-5.5281, 19.3836) (-5.5485, 19.4105) (-5.569, 19.4372) (-5.5897, 19.4639) (-5.6105, 19.4906) (-5.6315, 19.5172) (-5.6526, 19.5437) (-5.6739, 19.5702) (-5.6953, 19.5966) (-5.7168, 19.6229) (-5.7385, 19.6492) (-5.7603, 19.6754) (-5.7822, 19.7015) (-5.8043, 19.7276) (-5.8265, 19.7536) (-5.8488, 19.7796) (-5.8712, 19.8055) (-5.8938, 19.8314) (-5.9165, 19.8571) (-5.9394, 19.8829) (-5.9623, 19.9085) (-5.9854, 19.9341) (-6.0087, 19.9597) (-6.032, 19.9851) (-6.0555, 20.0106) (-6.079, 20.0359) (-6.098, 20.0562) (-6.1123, 20.0713) (-6.1218, 20.0814) (-6.1266, 20.0864) knots 0.195913 0.195913 0.195913 0.195913 0.195913 0.195913 0.2 0.214286 0.228571 0.242857 0.257143 0.271429 0.285714 0.3 0.314286 0.328571 0.342857 0.357143 0.371429 0.385714 0.4 0.414286 0.428571 0.442857 0.457143 0.471429 0.485714 0.5 0.514286 0.528571 0.542857 0.557143 0.571429 0.585714 0.6 0.614286 0.628571 0.642857 0.657143 0.671429 0.685714 0.7 0.714286 0.728571 0.742857 0.757143 0.771429 0.785714 0.8 0.814286 0.828571 0.842857 0.857143 0.871429 0.885714 0.9 0.914286 0.928571 0.942857 0.957143 0.971429 0.985714 1 1 1 1 1 1
  arc A65 (-6.1266, 20.0864) -> (-6.85, 19.8514) centre (0, 0) ccw
  spline S130 degree 5 poles (-6.85, 19.8514) (-6.8509, 19.8445) (-6.8527, 19.8307) (-6.8553, 19.8101) (-6.8588, 19.7826) (-6.863, 19.7482) (-6.867, 19.7138) (-6.8709, 19.6795) (-6.8747, 19.6452) (-6.8783, 19.6109) (-6.8818, 19.5767) (-6.8852, 19.5424) (-6.8884, 19.5082) (-6.8915, 19.474) (-6.8944, 19.4399) (-6.8972, 19.4057) (-6.8999, 19.3716) (-6.9024, 19.3376) (-6.9048, 19.3035) (-6.907, 19.2695) (-6.9091, 19.2355) (-6.911, 19.2015) (-6.9128, 19.1676) (-6.9144, 19.1337) (-6.9159, 19.0998) (-6.9173, 19.066) (-6.9185, 19.0322) (-6.9195, 18.9984) (-6.9204, 18.9647) (-6.9211, 18.931) (-6.9217, 18.8973) (-6.9221, 18.8637) (-6.9224, 18.8301) (-6.9224, 18.7966) (-6.9224, 18.7631) (-6.9221, 18.7296) (-6.9218, 18.6962) (-6.9212, 18.6628) (-6.9205, 18.6294) (-6.9195, 18.5961) (-6.9185, 18.5629) (-6.9172, 18.5296) (-6.9158, 18.4965) (-6.9142, 18.4634) (-6.9124, 18.4303) (-6.9104, 18.3973) (-6.9083, 18.3643) (-6.9059, 18.3314) (-6.9033, 18.2985) (-6.9006, 18.2657) (-6.8977, 18.233) (-6.8945, 18.2003) (-6.8912, 18.1676) (-6.8876, 18.1351) (-6.8838, 18.1026) (-6.8798, 18.0701) (-6.8756, 18.0378) (-6.8717, 18.0101) (-6.8687, 17.9889) (-6.8665, 17.9742) (-6.8652, 17.9659) (-6.8649, 17.9641) knots -1 -1 -1 -1 -1 -1 -0.985714 -0.971429 -0.957143 -0.942857 -0.928571 -0.914286 -0.9 -0.885714 -0.871429 -0.857143 -0.842857 -0.828571 -0.814286 -0.8 -0.785714 -0.771429 -0.757143 -0.742857 -0.728571 -0.714286 -0.7 -0.685714 -0.671429 -0.657143 -0.642857 -0.628571 -0.614286 -0.6 -0.585714 -0.571429 -0.557143 -0.542857 -0.528571 -0.514286 -0.5 -0.485714 -0.471429 -0.457143 -0.442857 -0.428571 -0.414286 -0.4 -0.385714 -0.371429 -0.357143 -0.342857 -0.328571 -0.314286 -0.3 -0.285714 -0.271429 -0.257143 -0.242857 -0.228571 -0.214286 -0.2 -0.195913 -0.195913 -0.195913 -0.195913 -0.195913 -0.195913
  spline S131 degree 3 poles (-7.1689, 17.426) (-7.1087, 17.4508) (-7.0539, 17.4871) (-6.9613, 17.5786) (-6.9244, 17.633) (-6.8809, 17.7354) (-6.8688, 17.7803) (-6.8573, 17.872) (-6.8579, 17.9184) (-6.8649, 17.9641) knots 0 0 0 0 0.019532 0.019532 0.039064 0.039064 0.052927 0.052927 0.06679 0.06679 0.06679 0.06679
  arc A66 (-7.1689, 17.426) -> (-7.2528, 17.3912) centre (0, 0) ccw
  spline S132 degree 3 poles (-7.8483, 17.5567) (-7.8098, 17.5043) (-7.7613, 17.4598) (-7.6502, 17.392) (-7.5885, 17.3693) (-7.4786, 17.3517) (-7.4322, 17.3507) (-7.3404, 17.3617) (-7.2955, 17.3734) (-7.2528, 17.3912) knots 0 0 0 0 0.019532 0.019532 0.039064 0.039064 0.052927 0.052927 0.06679 0.06679 0.06679 0.06679
  spline S133 degree 5 poles (-7.8483, 17.5567) (-7.8494, 17.5582) (-7.8544, 17.565) (-7.8632, 17.577) (-7.876, 17.5941) (-7.8929, 17.6164) (-7.9127, 17.6423) (-7.9329, 17.668) (-7.9532, 17.6937) (-7.9737, 17.7192) (-7.9944, 17.7447) (-8.0153, 17.77) (-8.0364, 17.7953) (-8.0576, 17.8204) (-8.079, 17.8455) (-8.1006, 17.8704) (-8.1224, 17.8952) (-8.1444, 17.92) (-8.1665, 17.9446) (-8.1888, 17.9692) (-8.2112, 17.9936) (-8.2338, 18.018) (-8.2566, 18.0423) (-8.2795, 18.0665) (-8.3026, 18.0906) (-8.3258, 18.1146) (-8.3491, 18.1385) (-8.3726, 18.1623) (-8.3963, 18.1861) (-8.4201, 18.2098) (-8.444, 18.2333) (-8.4681, 18.2568) (-8.4923, 18.2802) (-8.5166, 18.3035) (-8.5411, 18.3267) (-8.5657, 18.3499) (-8.5905, 18.3729) (-8.6153, 18.3959) (-8.6403, 18.4188) (-8.6655, 18.4416) (-8.6907, 18.4644) (-8.7161, 18.487) (-8.7416, 18.5096) (-8.7672, 18.532) (-8.793, 18.5544) (-8.8189, 18.5768) (-8.8449, 18.599) (-8.871, 18.6211) (-8.8972, 18.6432) (-8.9236, 18.6652) (-8.95, 18.6871) (-8.9766, 18.709) (-9.0033, 18.7307) (-9.0301, 18.7524) (-9.0571, 18.774) (-9.0841, 18.7955) (-9.1112, 18.8169) (-9.1385, 18.8383) (-9.1604, 18.8553) (-9.1769, 18.868) (-9.1879, 18.8765) (-9.1934, 18.8807) knots 0.195913 0.195913 0.195913 0.195913 0.195913 0.195913 0.2 0.214286 0.228571 0.242857 0.257143 0.271429 0.285714 0.3 0.314286 0.328571 0.342857 0.357143 0.371429 0.385714 0.4 0.414286 0.428571 0.442857 0.457143 0.471429 0.485714 0.5 0.514286 0.528571 0.542857 0.557143 0.571429 0.585714 0.6 0.614286 0.628571 0.642857 0.657143 0.671429 0.685714 0.7 0.714286 0.728571 0.742857 0.757143 0.771429 0.785714 0.8 0.814286 0.828571 0.842857 0.857143 0.871429 0.885714 0.9 0.914286 0.928571 0.942857 0.957143 0.971429 0.985714 1 1 1 1 1 1
  arc A67 (-9.1934, 18.8807) -> (-9.8711, 18.5354) centre (0, 0) ccw
  spline S134 degree 5 poles (-9.8711, 18.5354) (-9.8709, 18.5285) (-9.8705, 18.5146) (-9.8699, 18.4938) (-9.869, 18.4661) (-9.8678, 18.4315) (-9.8664, 18.3969) (-9.8649, 18.3624) (-9.8632, 18.3279) (-9.8614, 18.2935) (-9.8595, 18.2591) (-9.8575, 18.2247) (-9.8553, 18.1905) (-9.853, 18.1562) (-9.8506, 18.122) (-9.848, 18.0879) (-9.8453, 18.0538) (-9.8425, 18.0197) (-9.8395, 17.9857) (-9.8364, 17.9518) (-9.8331, 17.9179) (-9.8297, 17.884) (-9.8262, 17.8502) (-9.8225, 17.8165) (-9.8187, 17.7828) (-9.8147, 17.7492) (-9.8106, 17.7156) (-9.8063, 17.6821) (-9.8019, 17.6486) (-9.7974, 17.6152) (-9.7927, 17.5819) (-9.7878, 17.5486) (-9.7828, 17.5154) (-9.7777, 17.4822) (-9.7723, 17.4492) (-9.7669, 17.4161) (-9.7613, 17.3832) (-9.7555, 17.3503) (-9.7495, 17.3175) (-9.7434, 17.2847) (-9.7372, 17.252) (-9.7307, 17.2194) (-9.7241, 17.1869) (-9.7174, 17.1544) (-9.7104, 17.122) (-9.7033, 17.0897) (-9.696, 17.0575) (-9.6885, 17.0254) (-9.6809, 16.9933) (-9.673, 16.9613) (-9.665, 16.9295) (-9.6568, 16.8977) (-9.6484, 16.866) (-9.6397, 16.8343) (-9.6309, 16.8028) (-9.6219, 16.7714) (-9.6127, 16.7401) (-9.6045, 16.7134) (-9.5982, 16.6929) (-9.5937, 16.6788) (-9.5912, 16.6708) (-9.5906, 16.669) knots -1 -1 -1 -1 -1 -1 -0.985714 -0.971429 -0.957143 -0.942857 -0.928571 -0.914286 -0.9 -0.885714 -0.871429 -0.857143 -0.842857 -0.828571 -0.814286 -0.8 -0.785714 -0.771429 -0.757143 -0.742857 -0.728571 -0.714286 -0.7 -0.685714 -0.671429 -0.657143 -0.642857 -0.628571 -0.614286 -0.6 -0.585714 -0.571429 -0.557143 -0.542857 -0.528571 -0.514286 -0.5 -0.485714 -0.471429 -0.457143 -0.442857 -0.428571 -0.414286 -0.4 -0.385714 -0.371429 -0.357143 -0.342857 -0.328571 -0.314286 -0.3 -0.285714 -0.271429 -0.257143 -0.242857 -0.228571 -0.214286 -0.2 -0.195913 -0.195913 -0.195913 -0.195913 -0.195913 -0.195913
  spline S135 degree 3 poles (-9.8067, 16.09) (-9.7511, 16.1239) (-9.7026, 16.1683) (-9.6255, 16.2732) (-9.5976, 16.3327) (-9.5706, 16.4407) (-9.5657, 16.4869) (-9.5687, 16.5792) (-9.5765, 16.625) (-9.5906, 16.669) knots 0 0 0 0 0.019532 0.019532 0.039064 0.039064 0.052927 0.052927 0.06679 0.06679 0.06679 0.06679
  arc A68 (-9.8067, 16.09) -> (-9.8841, 16.0425) centre (0, 0) ccw
  spline S136 degree 3 poles (-10.4982, 16.1129) (-10.4519, 16.067) (-10.3971, 16.0307) (-10.2767, 15.9811) (-10.2122, 15.9683) (-10.1009, 15.9681) (-10.0549, 15.9745) (-9.966, 15.9996) (-9.9235, 16.0183) (-9.8841, 16.0425) knots 0 0 0 0 0.019532 0.019532 0.039064 0.039064 0.052927 0.052927 0.06679 0.06679 0.06679 0.06679